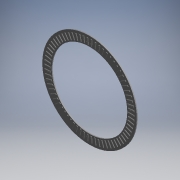
# Autodesk Inventor part: NTA-4860
Saved by Autodesk Inventor 2017.3 (Build 213256000, 256)
## iProperties
Part Number: NTA-4860
Material: Generic
Catalog Web Link: www.cadenas.de
Description: NTA, NTC Series-
Vendor: KOYO
Document SubType Name: Modeling
Designer: partserver
Manufacturer: KOYO
Mass: 3.05979 g
Surface Area: 61.4045 cm^2
Volume: 3.05979 cm^3
Density: 1 g/cm^3
Appearance: PSOLRGB-175-175-175
Category: PARTsolutions
Company: KOYO
Title: NTA-4860
Author: Cadenas PARTsolutions
PSOL_IDENT_0: {$CADENAS_DATA\23d-libs\koyo\needle_roller_bearings\needle_roller_thrust_bearings\inch_series\nta_nt
PSOL_IDENT_1: c_series.prj},166 {VTYP=3D},{NB=NTA-4860},{LINA=NTA-4860},{NN=NTA, NTC Series},{DATE=22.12.2017 04:3
PSOL_IDENT_2: 9:59},{GEOMDATE=24.03.2016 08:31:00},{VERSION=},{LINEID=230},{WBVAR=},{WBNUMERIC=}  {NB=NTA-4860},{L
PSOL_IDENT_3: INA=NTA-4860},{KT=DUMMY},{ORDER=NTA-4860},{SD=76.200},{D=95.250},{B=1.9837},{C=26.96},{CO=172.10},{C
PSOL_IDENT_4: U=17.60},{NO=4400},{E=78.490},{F=90.678},{S=NT},{T=10},{CB=0.99185},{ST=17-A},{NOB=70},{PDF=217}
NB: NTA-4860
NN: NTA, NTC Series
NBSYN: $ORDER.
LINA: NTA-4860
CATALOG: JTEKT Corporation(Koyo
ORDER: NTA-4860
SD: 76.2
D: 95.25
B: 1.9837
C: 26.96
CO: 172.1
CU: 17.6
NO: 4400
SUPPLIER: KOYO
ARTICLENO: NTA-4860
BOMINFO: NTA-4860
CREATOR: CADENAS GmbH
Autodesk Inventor part; units mm, degrees
ref_plane "YZ Plane" through (0, 0, 0) normal (1, 0, 0) x (0, 1, 0)
ref_plane "XZ Plane" through (0, 0, 0) normal (0, 1, 0) x (-1, 0, 0)
ref_plane "XY Plane" through (0, 0, 0) normal (0, 0, 1) x (1, 0, 0)
sketch "Sketch_1" plane through (0, 0, 0) normal (0, 0, 1) x (1, 0, 0)
  line L0 (0, 1.4878) -> (0, 0.4959)
  line L1 (-47.625, 1.4878) -> (-47.625, 0.4959)
  line L2 (-47.625, 0.4959) -> (-38.1, 0.4959)
  line L3 (-38.1, 0.4959) -> (-38.1, 1.4878)
  line L4 (-38.1, 1.4878) -> (-47.625, 1.4878)
  constraints: 10 end point
revolve "Revolution1" add sketch "Sketch_1" angle 360 about axis through (0, 1.4878, 0) along (0, 1, 0)
sketch "Sketch_4" plane through (0, 0.9919, 0) normal (0, 1, 0) x (1, 0, 0)
  line L0 (-39.245, 0) -> (-45.339, 0)
  line L1 (-45.339, 0) -> (-45.339, 0.9919)
  line L2 (-45.339, 0.9919) -> (-39.245, 0.9919)
  line L3 (-39.245, 0.9919) -> (-39.245, 0)
  line L4 (-39.245, 0) -> (-45.339, 0)
  constraints: 10 end point
revolve "Revolution2" add sketch "Sketch_4" angle 360 about axis through (-39.245, 0.9919, 0) along (1, 0, 0)
pattern_circular "Circular Pattern1" count 70 over 360 about axis through (0, 0.9919, 0) along (0, 1, 0) of "Revolution2"
body "Solid1"
